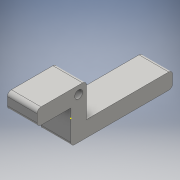
# Autodesk Inventor part: Lever
Saved by Autodesk Inventor 2016 (Build 200138000, 138)
## iProperties
Created: 2016-04-18
Part Number: Lever
Material: Generic
Document SubType Name: Modeling
Designer: amenoni
Density: 1 g/cm^3
Appearance: Default
Author: amenoni
Autodesk Inventor part; units mm, degrees
ref_plane "YZ Plane" through (0, 0, 0) normal (1, 0, 0) x (0, 1, 0)
ref_plane "XZ Plane" through (0, 0, 0) normal (0, 1, 0) x (-1, 0, 0)
ref_plane "XY Plane" through (0, 0, 0) normal (0, 0, 1) x (1, 0, 0)
sketch "Sketch1" plane through (0, 0, 0) normal (0, 1, 0) x (-1, 0, 0)
  line L0 (-7.5, -12.5) -> (7.5, -12.5)
  line L1 (7.5, -12.5) -> (7.5, 12.5)
  line L2 (7.5, 12.5) -> (-7.5, 12.5)
  line L3 (-7.5, 12.5) -> (-7.5, -12.5)
  line L4 (-7.5, -12.5) -> (7.5, 12.5) construction
  line L5 (7.5, -12.5) -> (-7.5, 12.5) construction
  point P0 (0, 0)
  dimension "d0" = 15
  dimension "d1" = 25
  constraints: 12 end point, 2 midpoint, 2 parallel, 1 horizontal, 1 perpendicular
  measures "d0" distance of L2.end L1.end
  measures "d1" distance of L1.end L0.end
extrude "Extrusion1" add sketch "Sketch1" along normal blind 8
sketch "Sketch2" plane through (7.5, 0, -12.5) normal (1, 0, 0) x (0, 0, -1)
  line L0 (-25, 0) -> (-25, 8) projected
  line L1 (-25, 8) -> (0, 8) projected
  point P0 (-12.5, 0)
  point P1 (-21, 4)
  point P2 (-25, 2)
  point P3 (-25, 6)
  point P4 (-23, 8)
  dimension "d5" = 4
  dimension "d6" = 4
  measures "d5" distance from line of L0 point (-21, 4)
  measures "d6" distance from line of L1 point (-21, 4)
hole "Hole1" at (7.5, 4, 8.5) direction (-1, 0, 0) diameter 4 end through all
sketch "Sketch4" plane through (7.5, 0, -12.5) normal (1, 0, 0) x (0, 0, -1)
  point P0 (-12.5, 0)
sketch "Sketch5" plane through (7.5, 0, 12.5) normal (1, 0, 0) x (0, 0, -1)
  line L0 (25, 0) -> (0, 0) projected
  line L1 (0, 0) -> (8, 0)
  line L2 (8, 0) -> (8, -17)
  line L3 (8, -17) -> (0, -17)
  line L4 (0, -17) -> (0, 0)
  point P0 (12.5, 0)
  dimension "d20" = 8
  dimension "d21" = 17
  constraints: 8 end point, 2 parallel, 1 horizontal, 1 perpendicular
  measures "d20" distance of L2.end L3.end
  measures "d21" distance of L1.end L2.end
extrude "Extrusion3" add sketch "Sketch5" against normal blind 15
fillet "Fillet3" radius 2 3 edges at (0, -17, 12.5) (0, -17, 4.5) (0, 8, 12.5)
sketch "Sketch6" plane through (7.5, 0, -12.5) normal (1, 0, 0) x (0, 0, -1)
  line L0 (0, 8) -> (-23, 8) projected
  line L1 (0, 8) -> (-8, 8)
  line L2 (-8, 8) -> (-8, 51.5)
  line L3 (-8, 51.5) -> (0, 51.5)
  line L4 (0, 51.5) -> (0, 8)
  point P0 (-12.5, 0)
  dimension "d25" = 8
  dimension "d26" = 43.5
  constraints: 8 end point, 2 parallel, 1 horizontal, 1 perpendicular
  measures "d25" distance of L2.end L3.end
  measures "d26" distance of L1.end L2.end
extrude "Extrusion4" add sketch "Sketch6" against normal blind 15
fillet "Fillet4" radius 2 3 edges at (0, 0, -12.5) (0, 51.5, -4.5) (0, 51.5, -12.5)
body "Solid1"
